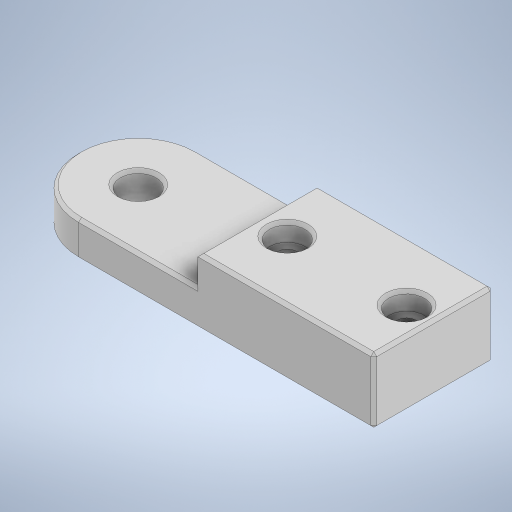
# Autodesk Inventor part: middle_joint
Saved by Autodesk Inventor 2023 (Build 270158000, 158)
## iProperties
Created: 2023-11-20
Part Number: middle_joint
Material: Všeobecné
Document SubType Name: Modeling
Designer: zavrel
Density: 1 g/cm^3
Appearance: Výchozí
Author: zavrel
Autodesk Inventor part; units mm, degrees
ref_plane "YZ Plane" through (0, 0, 0) normal (1, 0, 0) x (0, 1, 0)
ref_plane "XZ Plane" through (0, 0, 0) normal (0, 1, 0) x (-1, 0, 0)
ref_plane "XY Plane" through (0, 0, 0) normal (0, 0, 1) x (1, 0, 0)
sketch "Náčrt1" plane through (0, 0, 0) normal (0, 1, 0) x (-1, 0, 0)
  circle A0 centre (0, 0) radius 10
  line L0 (0, -10) -> (-50, -10)
  line L1 (-50, -10) -> (-50, 10)
  line L2 (-50, 10) -> (0, 10)
  circle A1 centre (0, 0) radius 3
  circle A2 centre (0, 0) radius 7.5 construction
  dimension "d0" = 6
  dimension "d1" = 15
  dimension "d2" = 20
  dimension "d3" = 50
  constraints: 6 end point, 3 centre point, 3 coincident, 2 perpendicular, 2 point on circle, 1 horizontal
  measures "d0" diameter of A1
  measures "d1" diameter of A2
  measures "d2" diameter of A0
  measures "d3" distance from line of L1 point (0, 0)
extrude "Vysunutí1" add sketch "Náčrt1" along normal blind 6
sketch "Náčrt2" plane through (0, 6, 0) normal (0, 1, 0) x (1, 0, 0)
  line L0 (0, -10) -> (50, -10) projected
  line L1 (50, -10) -> (50, 10) projected
  line L2 (50, 10) -> (0, 10) projected
  arc A0 (0, 10) -> (0, -10) centre (0, 0) ccw projected
  circle A1 centre (0, 0) radius 3 projected
  circle A2 centre (45, 0) radius 1.6
  circle A3 centre (25, 0) radius 1.6
  dimension "d6" = 5
  dimension "d7" = 25
  dimension "d8" = 3.2
  constraints: 2 centre point, 1 equal radius
  measures "d6" distance from line of L1 A2.centre
  measures "d7" distance from line of L1 A3.centre
  measures "d8" diameter of A3
extrude "Vysunutí2" cut sketch "Náčrt2" against normal through all contours A2 | A3
sketch "Náčrt5" plane through (0, 6, 0) normal (0, 1, 0) x (1, 0, 0)
  circle A0 centre (45, 0) radius 1.6 projected
  circle A1 centre (25, 0) radius 1.6 projected
  line L0 (0, -10) -> (50, -10) projected
  line L1 (50, -10) -> (50, 10) projected
  line L2 (50, 10) -> (0, 10) projected
  arc A2 (0, 10) -> (0, -10) centre (0, 0) ccw projected
  circle A3 centre (0, 0) radius 3 projected
  line L3 (20, 10) -> (20, -10)
  dimension "d19" = 30
  constraints: 2 end point, 2 point on line, 1 vertical
  measures "d19" distance between parallel lines of L1 L3
extrude "Vysunutí5" add sketch "Náčrt5" along normal blind 5 contours L3 L2 L1 L0
sketch "Náčrt7" plane through (0, 11, 0) normal (0, 1, 0) x (1, 0, 0)
  line L0 (50, 10) -> (20, 10) projected
  line L1 (20, 10) -> (20, -10) projected
  line L2 (20, -10) -> (50, -10) projected
  line L3 (50, -10) -> (50, 10) projected
  circle A0 centre (25, 0) radius 1.6 projected
  circle A1 centre (45, 0) radius 1.6 projected
  circle A2 centre (25, 0) radius 1.6 projected
  circle A3 centre (25, 0) radius 3
  circle A4 centre (45, 0) radius 1.6 projected
  circle A5 centre (45, 0) radius 3
  point P0 (0, 0)
  dimension "d22" = 6
  constraints: 2 centre point, 2 coincident, 1 equal radius
  measures "d22" diameter of A3
extrude "Vysunutí6" cut sketch "Náčrt7" against normal blind 3 contours A3 | A5
sketch "Náčrt8" plane through (50, 0, 10) normal (1, 0, 0) x (0, 0, -1)
  line L0 (0, 0) -> (20, 0) projected
  line L1 (20, 0) -> (20, 11) projected
  line L2 (0, 11) -> (20, 11) projected
  line L3 (0, 0) -> (0, 11) projected
  point P0 (10, 0)
extrude "Vysunutí7" cut sketch "Náčrt8" against normal blind 0.5
chamfer "Zkosení2" distance 0.5 angle 45 20 edges at (20, 11, 0) (22, 11, 0) (42, 11, 0) (24.75, 0, 10) (-10, 0, 0) (24.75, 0, -10) (10, 6, 10) (-10, 6, 0) (10, 6, -10) (34.75, 11, 10) (49.5, 11, 0) (34.75, 11, -10) (49.5, 0, 0) (49.5, 5.5, 10) (49.5, 5.5, -10) (3, 6, 0) (20, 6, 0) (3, 0, 0) (23.4, 0, 0) (43.4, 0, 0)
